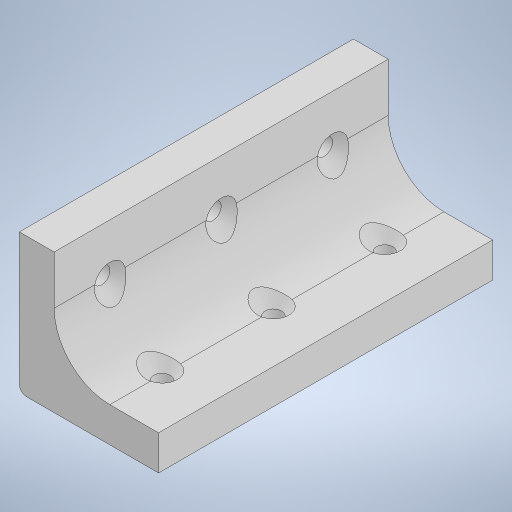
# Autodesk Inventor part: Arena Corner Bracket
Saved by Autodesk Inventor 2023.4 (Build 274418000, 418)
## iProperties
Created: 2024-04-25
Part Number: Arena Corner Bracket
Material: Generic
Document SubType Name: Modeling
Designer: Nathan Cai
Density: 1 g/cm^3
Appearance: Default
Author: Nathan Cai
Autodesk Inventor part; units mm, degrees
ref_plane "YZ Plane" through (0, 0, 0) normal (1, 0, 0) x (0, 1, 0)
ref_plane "XZ Plane" through (0, 0, 0) normal (0, 1, 0) x (-1, 0, 0)
sketch "Sketch1" plane through (0, 0, 0) normal (0, 0, 1) x (1, 0, 0)
  line L0 (0, 0) -> (7.9375, 0)
  line L1 (7.9375, 0) -> (7.9375, 31.75)
  line L2 (7.9375, 31.75) -> (0, 31.75)
  line L3 (0, 31.75) -> (0, 0)
  line L4 (0, 0) -> (31.75, 0)
  line L5 (31.75, 0) -> (31.75, 7.9375)
  line L6 (31.75, 7.9375) -> (0, 7.9375)
  line L7 (0, 7.9375) -> (0, 0)
  point P0 (7.9375, 7.9375)
  dimension "d0" = 7.9375
  dimension "d1" = 31.75
  dimension "d2" = 7.9375
  dimension "d3" = 31.75
  constraints: 16 end point, 4 parallel, 2 horizontal, 2 perpendicular
  measures "d0" distance of L2.end L1.end
  measures "d1" distance of L1.end L0.end
  measures "d2" distance of L4.end L5.end
  measures "d3" distance of L5.end L6.end
extrude "Extrusion1" add sketch "Sketch1" along normal blind 76.2
sketch "Sketch2" plane through (7.9375, 7.9375, 0) normal (1, 0, 0) x (0, 0, -1)
  line L0 (0, 0) -> (0, 23.8125) construction
  line L1 (0, 11.9062) -> (-76.2, 11.9063) construction
  line L2 (-76.2, 0) -> (-76.2, 23.8125) construction
  point P0 (0, -7.9375)
  point P1 (-12.7, 11.9063)
  point P2 (-38.1, 11.9063)
  point P3 (-63.5, 11.9063)
  dimension "d22" = 1.5875
  dimension "d7" = 12.7
  dimension "d10" = 25.4
  constraints: 2 end point, 2 midpoint, 1 horizontal, 1 point on line, 2 other
  measures "d7" distance from line of L0 point (-12.7, 11.906)
  measures "d10" distance of point (-12.7, 11.906) point (-38.1, 11.906)
hole "Hole1" at (7.9375, 19.8438, 12.7) at (7.9375, 19.8438, 38.1) at (7.9375, 19.8438, 63.5) direction (-1, 0, 0) diameter 3.81 end through all countersink diameter 7.0866 countersink angle 82 clearance for "Flat Head Machine Screw (82)" size "#6" standard "Ansi Unified Screw Threads"
ref_plane "Work Plane1" through (7.9375, 7.9375, 0) normal (0.7071068, -0.7071068, 0) x (0, 0, -1)
mirror "Mirror1" about plane through (7.9375, 7.9375, 0) normal (0.7071068, -0.7071068, 0) of "Hole1"
fillet "Fillet1" radius 12.7 1 edges at (7.9375, 7.9375, 38.1)
fillet "Fillet2" radius 1.5875 1 edges at (0, 0, 38.1)
equation "\"d2\" = d0"
equation "\"d3\" = d1"
body "Solid1"
